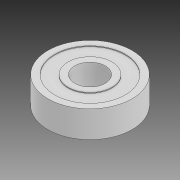
# Autodesk Inventor part: 608zz
Saved by Autodesk Inventor 2020 (Build 240168000, 168)
## iProperties
Created: 2020-09-16
Part Number: 608zz
Material: Generic
Document SubType Name: Modeling
Designer: DDeGo
Density: 1 g/cm^3
Appearance: Default
Author: DDeGo
Autodesk Inventor part; units mm, degrees
ref_plane "YZ Plane" through (0, 0, 0) normal (1, 0, 0) x (0, 1, 0)
ref_plane "XZ Plane" through (0, 0, 0) normal (0, 1, 0) x (-1, 0, 0)
ref_plane "XY Plane" through (0, 0, 0) normal (0, 0, 1) x (1, 0, 0)
sketch "Sketch1" plane through (0, 0, 0) normal (1, 0, 0) x (0, 1, 0)
  line L0 (0, 0) -> (7, 0) construction
  line L1 (7, 0) -> (7, -4) construction
  line L2 (7, -4) -> (0, -4)
  line L3 (0, -4) -> (0, 0) construction
  line L4 (7, -4) -> (7, -5.75)
  line L5 (7, -5.75) -> (6.8, -5.75)
  line L6 (6.8, -5.75) -> (6.8, -9.25)
  line L7 (6.8, -9.25) -> (7, -9.25)
  line L8 (7, -9.25) -> (7, -11)
  line L9 (7, -11) -> (0, -11)
  line L10 (0, -11) -> (0, -9.25)
  line L11 (0, -9.25) -> (0.2, -9.25)
  line L12 (0.2, -9.25) -> (0.2, -5.75)
  line L13 (0.2, -5.75) -> (0, -5.75)
  line L14 (0, -4) -> (0, -5.75)
  dimension "d0" = 4
  dimension "d1" = 11
  dimension "d2" = 7
  dimension "d3" = 0.2
  dimension "d4" = 3.5
  constraints: 30 end point, 10 perpendicular, 8 point on line, 3 collinear, 1 horizontal
  measures "d0" distance between parallel lines of L0 L2
  measures "d1" distance between parallel lines of L0 L9
  measures "d2" distance of L8.end L9.end
  measures "d3" distance between parallel lines of L4 L6
  measures "d4" distance of L5.end L6.end
revolve "Revolution1" add sketch "Sketch1" angle 360 about axis through (0, 0, 0) along (0, 1, 0)
body "Solid1"
